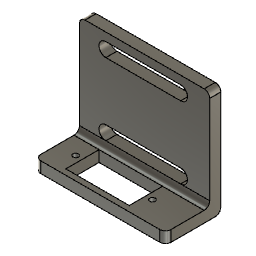
SOAR_Sensor_Holder-v1 (Autodesk Fusion 360 design; units mm, degrees)
Autodesk Fusion 360 part; units mm, degrees
sketch "Sketch1" plane through (0, 0, 0) normal (0, 0, 1) x (1, 0, 0)
  line L0 (31.95, 2) -> (31.95, 14)
  line L1 (0, 20) -> (0, 0)
  line L2 (47, 0) -> (47, 20)
  line L3 (4.25, 2) -> (4.25, 14)
  line L4 (47, 16) -> (0, 16)
  line L5 (4.25, 14) -> (36.75, 14)
  line L6 (0, 16) -> (0, 20)
  line L7 (36.75, 14) -> (36.75, 2)
  line L8 (47, 20) -> (47, 16)
  line L9 (4.25, 14) -> (4.25, 2)
  line L10 (36.75, 2) -> (4.25, 2)
  line L11 (47, 20) -> (0, 20)
  line L12 (0, 0) -> (47, 0)
  circle A0 centre (34.35, 8) radius 1
  circle A1 centre (6.65, 8) radius 1
  line L13 (4.25, 2) -> (9.05, 2)
  line L14 (36.75, 14) -> (36.75, 2)
  line L15 (31.95, 14) -> (36.75, 14)
  line L16 (9.05, 14) -> (4.25, 14)
  line L17 (9.05, 2) -> (9.05, 14)
  line L18 (0, 20) -> (47, 20)
  line L19 (36.75, 2) -> (31.95, 2)
  dimension "d1" = 47
  dimension "d2" = 20
  dimension "d5" = 4
  dimension "d20" = 32.5
  dimension "d21" = 12
  dimension "d22" = 4.8
  dimension "d23" = 4.8
  dimension "d24" = 2
  dimension "d25" = 2
  constraint horizontal L12
  constraint vertical L2
  constraint horizontal L11
  constraint vertical L1
  constraint coincident L1.end L12.start
  constraint horizontal L18
  constraint vertical L8
  constraint horizontal L4
  constraint vertical L6
  constraint horizontal L5
  constraint vertical L14
  constraint horizontal L10
  constraint vertical L3
  constraint horizontal L13
  constraint vertical L17
  constraint horizontal L16
  constraint vertical L9
  constraint coincident L16.start L5
  constraint horizontal L19
  constraint vertical L0
  constraint horizontal L15
  constraint vertical L7
  measures "d1" distance of L2.start L1.end
  measures "d2" distance of L1.end L1.start
  measures "d5" distance of L1.start L4.end
  measures "d20" distance of L5.end L3.end
  measures "d21" distance of L3.end L3.start
  measures "d22" distance of L13.end L3.start
  measures "d23" distance of L7.end L0.start
  measures "d24" diameter of A1
  measures "d25" diameter of A0
extrude "Extrude1" add sketch "Sketch1" along normal blind 4 contours L0 L5 L7 L10 L14 L15 L19 | L3 L5 L9 L10 L13 L16 L17 | L1 L2 L4 L12
extrude "Extrude2" add sketch "Sketch1" along normal blind 28 contours L1 L2 L4 L6 L8 L11 L18
extrude "Extrude3" add 1 faces at (15.6667, 18.6667, 28) along direction (0, 0, 1) blind 12
ref_plane "WorkPlane1" through (23.5, 18, 37) normal (0, 0, 1) x (1, 0, 0)
sketch "Sketch2" plane through (20, 18, 37) normal (0, 0, 1) x (1, 0, 0)
  line L0 (-13, -3) -> (19, -3)
  line L1 (19, -3) -> (19, 5)
  line L2 (19, 5) -> (-13, 5)
  line L3 (-13, 5) -> (-13, -3)
  constraint horizontal L0
  constraint vertical L1
  constraint horizontal L2
  constraint vertical L3
extrude "Extrude4" cut sketch "Sketch2" against normal blind 5
ref_plane "WorkPlane2" through (23, 18, 11) normal (0, 0, 1) x (1, 0, 0)
sketch "Sketch3" plane through (20, 18, 11) normal (0, 0, 1) x (1, 0, 0)
  line L0 (-13, -3) -> (19, -3)
  line L1 (19, -3) -> (19, 5)
  line L2 (19, 5) -> (-13, 5)
  line L3 (-13, 5) -> (-13, -3)
  constraint horizontal L0
  constraint vertical L1
  constraint horizontal L2
  constraint vertical L3
extrude "Extrude5" cut sketch "Sketch3" against normal blind 5
fillet "Fillet1" radius 2.5 8 edges at (7, 18, 6) (7, 18, 11) (39, 18, 11) (39, 18, 6) (39, 18, 32) (39, 18, 37) (7, 18, 37) (7, 18, 32)
fillet "Fillet2" radius 2 6 edges at (47, 18, 40) (0, 18, 40) (23.5, 16, 4) (47, 0, 2) (0, 0, 2) (23.5, 20, 0)
